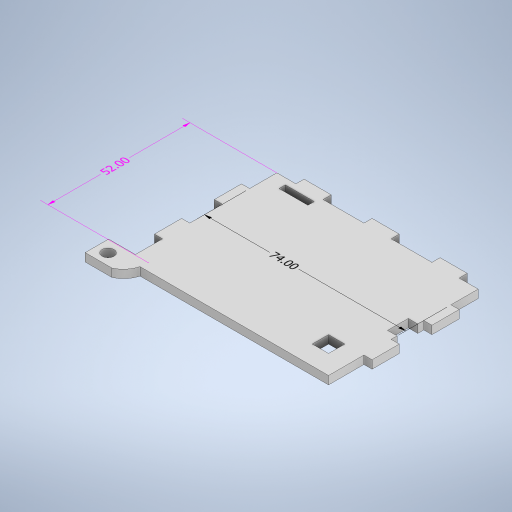
# Autodesk Inventor part: Parede_HX711
Saved by Autodesk Inventor 2024 (Build 280153000, 153)
## iProperties
Created: 2023-11-29
Part Number: Parede_HX711
Material: Genérico
Document SubType Name: Modeling
Designer: caiot
Density: 1 g/cm^3
Appearance: Padrão
Author: caiot
Autodesk Inventor part; units mm, degrees
ref_plane "YZ Plane" through (0, 0, 0) normal (1, 0, 0) x (0, 1, 0)
ref_plane "XZ Plane" through (0, 0, 0) normal (0, 1, 0) x (-1, 0, 0)
ref_plane "XY Plane" through (0, 0, 0) normal (0, 0, 1) x (1, 0, 0)
sketch "Esboço1" plane through (0, 0, 0) normal (0, 1, 0) x (-1, 0, 0)
  line L0 (0, 0) -> (-74, 0)
  line L1 (-74, 0) -> (-74, -52)
  line L2 (-74, -52) -> (0, -52)
  line L3 (0, -52) -> (0, 0)
  line L4 (-6.0465, -39.0348) -> (-22.7965, -39.0348)
  line L5 (-22.7965, -39.0348) -> (-22.7965, -36.6698)
  line L6 (-22.7965, -36.6698) -> (-6.0465, -36.6698)
  line L7 (-6.0465, -36.6698) -> (-6.0465, -39.0348)
  dimension "d0" = 74
  dimension "d1" = 52
  dimension "d22" = 16.75
  dimension "d23" = 2.365
  constraints: 16 end point, 4 parallel, 2 horizontal, 2 perpendicular
  measures "d0" distance of L2.end L1.end
  measures "d1" distance of L1.end L0.end
  measures "d22" distance of L5.end L6.end
  measures "d23" distance of L4.end L5.end
extrude "Extrusão1" add sketch "Esboço1" along normal blind 3 contours L3 L2 L1 L0 | L4 L5 L6 L7
sketch "Esboço2" plane through (0, 3, 0) normal (0, 1, 0) x (1, 0, 0)
  line L0 (0, 0) -> (74, 0) projected
  line L1 (0, 52) -> (0, 0) projected
  line L2 (74, 52) -> (0, 52) projected
  line L3 (7, 52) -> (17, 52)
  line L4 (17, 52) -> (17, 55)
  line L5 (17, 55) -> (7, 55)
  line L6 (7, 55) -> (7, 52)
  line L7 (32, 52) -> (42, 52)
  line L8 (42, 52) -> (42, 55)
  line L9 (42, 55) -> (32, 55)
  line L10 (32, 55) -> (32, 52)
  line L11 (57, 52) -> (67, 52)
  line L12 (67, 52) -> (67, 55)
  line L13 (67, 55) -> (57, 55)
  line L14 (57, 55) -> (57, 52)
  line L15 (74, 0) -> (74, 52) projected
  point P0 (17, 52)
  point P1 (67, 52)
  point P2 (42, 52)
  point P3 (74, 26)
  point P4 (32, 53.5)
  point P5 (17, 53.5)
  point P6 (7, 53.5)
  point P7 (67, 53.5)
  point P8 (42, 53.5)
  point P9 (57, 53.5)
  dimension "d13" = 3
  dimension "d40" = 7
  dimension "d41" = 7
  dimension "d43" = 10
  dimension "d46" = 10
  dimension "d52" = 10
  dimension "d54" = 40
  dimension "d55" = 15
  constraints: 24 end point, 7 midpoint, 6 parallel, 5 point on line, 3 horizontal, 3 perpendicular
  measures "d13" distance of L4.end L3.end
  measures "d40" distance from line of L1 point (7, 53.5)
  measures "d41" distance from line of L15 point (67, 53.5)
  measures "d43" distance of L9.end L8.end
  measures "d46" horizontal distance of L12.end L11.start
  measures "d52" distance of point (7, 53.5) point (17, 53.5)
  measures "d54" distance of point (57, 53.5) point (17, 53.5)
  measures "d55" distance of point (57, 53.5) point (42, 53.5)
extrude "Extrusão2" add sketch "Esboço2" against normal blind 3 contours L6 L5 L4 L2 | L2 L14 L13 L12 | L10 L9 L8 L2
sketch "Esboço4" plane through (0, 0, 0) normal (0, -1, 0) x (1, 0, 0)
  line L0 (16.0248, -49.74) -> (5.3998, -49.74)
  line L1 (5.3998, -49.74) -> (5.3998, -47.39)
  line L2 (5.3998, -47.39) -> (16.0248, -47.39)
  line L3 (16.0248, -47.39) -> (16.0248, -49.74)
  line L4 (7, -52) -> (0, -52) projected
  point P0 (0, 0)
  dimension "d24" = 10.625
  dimension "d25" = 2.35
  dimension "d120" = 2.26
  constraints: 8 end point, 2 parallel, 1 horizontal, 1 perpendicular
  measures "d24" distance of L1.end L2.end
  measures "d25" distance of L0.end L1.end
  measures "d120" distance between parallel lines of L4 L0
extrude "Extrusão3" cut sketch "Esboço4" against normal blind 3
sketch "Esboço5" plane through (0, 3, 0) normal (0, 1, 0) x (1, 0, 0)
  line L0 (70.5, 22.2) -> (74, 22.2)
  line L1 (74, 22.2) -> (74, 29.8)
  line L2 (74, 29.8) -> (70.5, 29.8)
  line L3 (70.5, 29.8) -> (70.5, 22.2)
  line L4 (74, 0) -> (74, 52) projected
  line L5 (74, 52) -> (67, 52) projected
  point P0 (0, 0)
  point P1 (74, 26)
  point P2 (72.25, 29.8)
  dimension "d47" = 3.5
  dimension "d48" = 7.6
  dimension "d51" = 0
  dimension "d79" = 22.2
  constraints: 8 end point, 2 midpoint, 2 parallel, 1 horizontal, 1 perpendicular
  measures "d47" distance of L2.end L1.end
  measures "d48" distance of L1.end L0.end
  measures "d51" distance from line of L4 point (74, 26)
  measures "d79" distance from line of L5 point (72.25, 29.8)
extrude "Extrusão4" cut sketch "Esboço5" against normal blind 10
sketch "Esboço6" plane through (0, 3, 0) normal (0, 1, 0) x (1, 0, 0)
  line L0 (0, 10) -> (-3, 10)
  line L1 (-3, 10) -> (-3, 20)
  line L2 (-3, 20) -> (0, 20)
  line L3 (0, 20) -> (0, 10)
  line L4 (0, 32) -> (-3, 32)
  line L5 (-3, 32) -> (-3, 42)
  line L6 (-3, 42) -> (0, 42)
  line L7 (0, 42) -> (0, 32)
  line L8 (7, 52) -> (0, 52) projected
  line L9 (0, 0) -> (74, 0) projected
  line L10 (74, 52) -> (67, 52) projected
  line L11 (0, 0) -> (74, 0) projected
  line L12 (74, 0) -> (74, 22.2) projected
  line L13 (74, 10) -> (77, 10)
  line L14 (77, 10) -> (77, 20)
  line L15 (77, 20) -> (74, 20)
  line L16 (74, 20) -> (74, 10)
  line L17 (74, 29.8) -> (74, 52) projected
  line L18 (74, 32) -> (77, 32)
  line L19 (77, 32) -> (77, 42)
  line L20 (77, 42) -> (74, 42)
  line L21 (74, 42) -> (74, 32)
  point P0 (-1.5, 42)
  point P1 (7, 0)
  point P2 (-1.5, 10)
  point P3 (67, 0)
  point P4 (75.5, 10)
  dimension "d62" = 3
  dimension "d63" = 10
  dimension "d64" = 3
  dimension "d65" = 10
  dimension "d66" = 10
  dimension "d67" = 10
  dimension "d74" = 3
  dimension "d75" = 10
  dimension "d76" = 10
  constraints: 32 end point, 8 parallel, 4 horizontal, 4 perpendicular, 3 midpoint, 3 point on line
  measures "d62" distance of L1.end L2.end
  measures "d63" distance of L0.end L1.end
  measures "d64" distance of L5.end L6.end
  measures "d65" distance of L4.end L5.end
  measures "d66" distance from line of L8 point (-1.5, 42)
  measures "d67" distance from line of L9 point (-1.5, 10)
  measures "d74" distance of L15.end L14.end
  measures "d75" distance of L14.end L13.end
  measures "d76" distance from line of L11 point (75.5, 10)
extrude "Extrusão5" add sketch "Esboço6" against normal blind 3
sketch "Esboço8" plane through (0, 0, 0) normal (0, -1, 0) x (1, 0, 0)
  line L0 (0, 0) -> (74, 0) projected
  line L1 (4.9609, 0) -> (-9.8465, 0)
  line L2 (-9.8465, 0) -> (-9.8465, 8.6)
  line L3 (0, -10) -> (0, 0) projected
  circle A0 centre (-5.5465, 4.4971) radius 2.2
  line L4 (-9.8465, 8.6) -> (0, 8.6)
  line L5 (0, 8.6) -> (0, 0)
  line L6 (0, 0) -> (-9.8465, 0)
  line L7 (-9.8465, 0) -> (-9.8465, 8.6)
  arc A1 (4.9609, 0) -> (0, 8.6) centre (-3.4963, 0.8523) ccw
  point P0 (0, 4.3)
  point P1 (-4.9233, 8.6)
  dimension "d100" = 8.6
  dimension "d102" = 4.4
  dimension "d104" = 4.3
  dimension "d121" = 8.5
  dimension "d123" = 4.15
  dimension "d124" = 5.55
  dimension "d128" = 9.8465
  dimension "d130" = 9.8465
  constraints: 12 end point, 2 centre point, 2 horizontal, 2 midpoint, 2 parallel, 2 perpendicular, 2 point on circle, 1 point on line
  measures "d100" distance of L1.end L2.end
  measures "d102" diameter of A0
  measures "d104" distance from line of L2 A0.centre
  measures "d121" radius of A1
  measures "d123" distance of point (-4.923, 8.6) A0.centre
  measures "d124" distance of point (0, 4.3) A0.centre
  measures "d128" distance between parallel lines of L5 L2
  measures "d130" distance between parallel lines of L3 L2
extrude "Extrusão7" add sketch "Esboço8" against normal blind 3
sketch "Esboço11" plane through (0, 0, 0) normal (0, -1, 0) x (1, 0, 0)
  line L0 (0, 0) -> (74, 0)
  line L1 (74, 0) -> (74, 3)
  line L2 (74, 3) -> (0, 3)
  line L3 (0, 3) -> (0, 0)
  dimension "d129" = 3
  constraints: 8 end point, 2 parallel, 1 horizontal, 1 perpendicular
  measures "d129" distance of L1.end L0.end
extrude "Extrusão9" add sketch "Esboço11" against normal blind 3
sketch "Esboço12" plane through (0, 3, 0) normal (0, 1, 0) x (1, 0, 0)
  line L0 (67, 4) -> (61, 4)
  line L1 (61, 4) -> (61, 10)
  line L2 (61, 10) -> (67, 10)
  line L3 (67, 10) -> (67, 4)
  line L4 (4.728, -3) -> (74, -3) projected
  line L5 (74, -3) -> (74, 10) projected
  line L6 (74, 10) -> (77, 10) projected
  point P0 (0, 0)
  point P1 (64, 4)
  point P2 (67, 7)
  point P3 (75.5, 10)
  dimension "d131" = 6
  dimension "d132" = 6
  dimension "d134" = 7
  dimension "d135" = 0
  constraints: 8 end point, 3 midpoint, 2 parallel, 1 horizontal, 1 perpendicular
  measures "d131" distance of L1.end L2.end
  measures "d132" distance of L0.end L1.end
  measures "d134" distance from line of L5 point (67, 7)
  measures "d135" distance from line of point (75.5, 10) L2
extrude "Extrusão10" cut sketch "Esboço12" against normal blind 10
equation "\"d55\" = -0.5 * d43 + 0.5 * d54"
